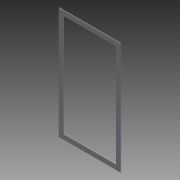
# Autodesk Inventor part: inside lining
Saved by Autodesk Inventor 2012 (Build 160160000, 160)
## iProperties
Created: 2012-04-20
Part Number: inside lining
Material: Default
Document SubType Name: Modeling
Designer: Puzzles
Density: 1 g/cm^3
Author: Puzzles
Autodesk Inventor part; units mm, degrees
ref_plane "YZ Plane" through (0, 0, 0) normal (1, 0, 0) x (0, 1, 0)
ref_plane "XZ Plane" through (0, 0, 0) normal (0, 1, 0) x (-1, 0, 0)
ref_plane "XY Plane" through (0, 0, 0) normal (0, 0, 1) x (1, 0, 0)
sketch "Sketch1" plane through (0, 0, 0) normal (0, 0, 1) x (1, 0, 0)
  line L0 (-165.1, 298.45) -> (165.1, 298.45)
  line L1 (165.1, 298.45) -> (165.1, -298.45)
  line L2 (165.1, -298.45) -> (-165.1, -298.45)
  line L3 (-165.1, -298.45) -> (-165.1, 298.45)
  point P0 (0, 0)
  point P1 (0, 298.45)
  point P2 (-165.1, 0)
  dimension "d0" = 330.2
  dimension "d1" = 596.9
  constraints: 8 end point, 2 midpoint, 2 parallel, 1 horizontal, 1 horizontal alignment, 1 perpendicular, 1 vertical alignment
  measures "d0" distance of L0.start L0.end
  measures "d1" distance of L2.end L0.start
extrude "Extrusion1" add sketch "Sketch1" along normal blind 3
sketch "Sketch2" plane through (0, 0, 3) normal (0, 0, 1) x (1, 0, 0)
  line L0 (165.1, 298.45) -> (165.1, -298.45) projected
  line L1 (-165.1, 298.45) -> (165.1, 298.45) projected
  line L2 (-165.1, -298.45) -> (-165.1, 298.45) projected
  line L3 (165.1, -298.45) -> (-165.1, -298.45) projected
  line L4 (-139.7, 273.05) -> (139.7, 273.05)
  line L5 (139.7, 273.05) -> (139.7, -273.05)
  line L6 (139.7, -273.05) -> (-139.7, -273.05)
  line L7 (-139.7, -273.05) -> (-139.7, 273.05)
  point P0 (0, 0)
  dimension "d4" = 25.4
  dimension "d5" = 25.4
  dimension "d6" = 25.4
  dimension "d7" = 25.4
  constraints: 8 end point, 2 parallel, 1 horizontal, 1 perpendicular
  measures "d4" distance between parallel lines of L3 L6
  measures "d5" distance between parallel lines of L2 L7
  measures "d6" distance between parallel lines of L0 L5
  measures "d7" distance between parallel lines of L1 L4
extrude "Extrusion2" cut sketch "Sketch2" against normal blind 3 contours L4 L5 L6 L7
body "Solid1"
